x_tensioner (Autodesk Fusion 360 design; units mm, degrees)
Autodesk Fusion 360 part; units mm, degrees
sketch "Sketch1" plane through (0, 0, 0) normal (1, 0, 0) x (0, 0, -1)
  line L0 (0, 0) -> (19, 0)
  line L1 (19, 0) -> (19, 60)
  line L2 (19, 60) -> (0, 60)
  line L3 (0, 60) -> (0, 0)
  circle A0 centre (9.5, 52.5) radius 1.65
  circle A1 centre (9.5, 7.5) radius 1.65
  circle A2 centre (9.5, 30) radius 2.1
  point P0 (9.5, 60)
  point P1 (0, 30)
  dimension "d1" = 3.3
  dimension "d2" = 45
  dimension "d3" = 60
  dimension "d4" = 19
  dimension "d5" = 9.5
  dimension "d6" = 7.5
  dimension "d7" = 4.2
  constraint horizontal L0
  constraint vertical L1
  constraint horizontal L2
  constraint vertical L3
  constraint coincident L0.start L3.end
  constraint equal A0 A1
  constraint vertical A0.centre A1.centre
  constraint midpoint L2 P0
  constraint midpoint L3 P1
  constraint horizontal A2.centre P1
  constraint vertical A2.centre P0
  measures "d1" diameter of A1
  measures "d2" distance of A0.centre A1.centre
  measures "d3" distance of L0.start L2.end
  measures "d4" distance of L1.end L2.end
  measures "d5" distance of L1 A0.centre
  measures "d6" distance of L2 A0.centre
  measures "d7" diameter of A2
extrude "Extrude1" add sketch "Sketch1" along normal blind 4
sketch "Sketch2" plane through (4, 0, 0) normal (1, 0, 0) x (0, 0, -1)
  circle A0 centre (9.5, 7.5) radius 1.65
  circle A1 centre (9.5, 52.5) radius 1.65
  circle A2 centre (9.5, 30) radius 2.1
  line L0 (0, 60) -> (0, 0)
  line L1 (0, 0) -> (19, 0)
  line L2 (19, 0) -> (19, 60)
  line L3 (19, 60) -> (0, 60)
  line L4 (19, 40.5) -> (0, 40.5)
  line L5 (0, 40.5) -> (0, 19.5)
  line L6 (0, 19.5) -> (19, 19.5)
  line L7 (19, 19.5) -> (19, 40.5)
  line L8 (19, 40.5) -> (0, 19.5) construction
  line L9 (0, 40.5) -> (19, 19.5) construction
  point P0 (9.5, 30)
  dimension "d10" = 21
  constraint horizontal L4
  constraint perpendicular L4 L5
  constraint parallel L4 L6
  constraint parallel L5 L7
  constraint coincident L2 L4.start
  constraint coincident L8 P0
  constraint coincident L9 P0
  constraint coincident P0 A2.centre
  measures "d10" distance of L4 L6
extrude "Extrude2" cut sketch "Sketch2" against normal blind 1 contours L0 L2 L4 L5 L6 L7
fillet "Fillet1" radius 3 4 edges at (2, 60, 0) (2, 60, -19) (2, 0, -19) (2, 0, 0)
sketch "Sketch3" plane through (0, 0, 0) normal (-1, 0, 0) x (0, 0, 1)
  arc A0 (-3, 0) -> (0, 3) centre (-3, 3) ccw
  line L0 (0, 3) -> (0, 57)
  arc A1 (0, 57) -> (-3, 60) centre (-3, 57) ccw
  line L1 (-3, 60) -> (-16, 60)
  arc A2 (-16, 60) -> (-19, 57) centre (-16, 57) ccw
  line L2 (-19, 57) -> (-19, 3)
  arc A3 (-19, 3) -> (-16, 0) centre (-16, 3) ccw
  line L3 (-16, 0) -> (-3, 0)
  circle A4 centre (-9.5, 7.5) radius 1.65
  circle A5 centre (-9.5, 52.5) radius 1.65
  circle A6 centre (-9.5, 30) radius 2.1
  line L4 (-11.2321, 55.5) -> (-12.9641, 52.5)
  line L5 (-12.9641, 52.5) -> (-11.2321, 49.5)
  line L6 (-11.2321, 49.5) -> (-7.7679, 49.5)
  line L7 (-7.7679, 49.5) -> (-6.0359, 52.5)
  line L8 (-6.0359, 52.5) -> (-7.7679, 55.5)
  line L9 (-7.7679, 55.5) -> (-11.2321, 55.5)
  line L10 (-11.2321, 10.5) -> (-12.9641, 7.5)
  line L11 (-12.9641, 7.5) -> (-11.2321, 4.5)
  line L12 (-11.2321, 4.5) -> (-7.7679, 4.5)
  line L13 (-7.7679, 4.5) -> (-6.0359, 7.5)
  line L14 (-6.0359, 7.5) -> (-7.7679, 10.5)
  line L15 (-7.7679, 10.5) -> (-11.2321, 10.5)
  point P0 (-9.5, 52.5)
  point P1 (-9.5, 7.5)
  dimension "d15" = 6
  dimension "d16" = 6
  constraint coincident P0 A5.centre
  constraint coincident P1 A4.centre
  constraint horizontal L9
  constraint horizontal L15
  measures "d15" distance of L12 L15
  measures "d16" distance of L6 L9
extrude "Extrude3" cut sketch "Sketch3" against normal blind 3 contours L4 L5 L6 L7 L8 L9 | L10 L11 L12 L13 L14 L15
equation "d5 = d4 / 2"
equation "d16 = d15"
